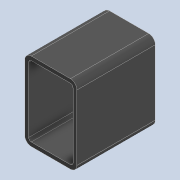
# Autodesk Inventor part: Generic 2x3in Steel Square Tubing
Saved by Autodesk Inventor 2022 (Build 260153000, 153)
## iProperties
Created: 2021-10-10
Part Number: Generic 2x3in Steel Square Tubing
Material: Generic
Document SubType Name: Modeling
Designer: Coy
Density: 1 g/cm^3
Appearance: Generic
Author: Coy
Autodesk Inventor part; units mm, degrees
ref_plane "YZ Plane" through (0, 0, 0) normal (1, 0, 0) x (0, 1, 0)
ref_plane "XZ Plane" through (0, 0, 0) normal (0, 1, 0) x (-1, 0, 0)
ref_plane "XY Plane" through (0, 0, 0) normal (0, 0, 1) x (1, 0, 0)
sketch "Sketch1" plane through (0, 0, 0) normal (0, 0, 1) x (1, 0, 0)
  line L0 (6.35, 0) -> (44.45, 0)
  line L1 (50.8, 6.35) -> (50.8, 69.85)
  line L2 (44.45, 76.2) -> (6.35, 76.2)
  line L3 (0, 69.85) -> (0, 6.35)
  arc A0 (6.35, 76.2) -> (0, 69.85) centre (6.35, 69.85) ccw
  arc A1 (50.8, 69.85) -> (44.45, 76.2) centre (44.45, 69.85) ccw
  arc A2 (44.45, 0) -> (50.8, 6.35) centre (44.45, 6.35) ccw
  arc A3 (0, 6.35) -> (6.35, 0) centre (6.35, 6.35) ccw
  line L4 (3.81, 69.85) -> (3.81, 6.35)
  arc A4 (3.81, 6.35) -> (6.35, 3.81) centre (6.35, 6.35) ccw
  line L5 (6.35, 3.81) -> (44.45, 3.81)
  arc A5 (44.45, 3.81) -> (46.99, 6.35) centre (44.45, 6.35) ccw
  line L6 (46.99, 6.35) -> (46.99, 69.85)
  arc A6 (46.99, 69.85) -> (44.45, 72.39) centre (44.45, 69.85) ccw
  line L7 (44.45, 72.39) -> (6.35, 72.39)
  arc A7 (6.35, 72.39) -> (3.81, 69.85) centre (6.35, 69.85) ccw
  point P0 (0, 0)
  point P1 (50.8, 76.2)
  point P2 (50.8, 0)
  point P3 (0, 76.2)
  dimension "d0" = 50.8
  dimension "d1" = 76.2
  dimension "d2" = 6.35
  dimension "d3" = 6.35
  dimension "d4" = 3.81
  constraints: 16 end point, 16 point on circle, 8 centre point, 8 point on line, 8 tangent, 4 parallel, 2 equal radius, 2 perpendicular, 1 horizontal, 7 other
  measures "d0" distance of point (0, 76.2) point (50.8, 76.2)
  measures "d1" distance of point (50.8, 76.2) point (50.8, 0)
  measures "d2" radius of A0
  measures "d3" radius of A3
  measures "d4" radial gap between concentric circles of A0 A7
extrude "Extrusion1" add sketch "Sketch1" along normal blind 76.2
body "Solid1"
